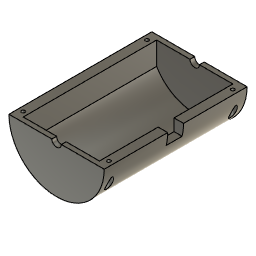
ShellTop (Autodesk Fusion 360 design; units mm, degrees)
Autodesk Fusion 360 part; units mm, degrees
note: some values were not read from the file. Set by a fixed rule: which sketch regions a step uses.
sketch "Sketch1" plane through (0, 0, 0) normal (0, 1, 0) x (1, 0, 0)
  circle A0 centre (38.1, -38.1) radius 38.1
  circle A1 centre (38.1, -38.1) radius 35.56
  circle A2 centre (38.1, -38.1) radius 3.81
  line L0 (38.1, -38.1) -> (0, -38.1)
  line L1 (38.1, -38.1) -> (76.2, -38.1)
  dimension "d1" = 76.2
  dimension "d2" = 71.12
  dimension "d4" = 7.62
  constraint concentric A0 A1
  constraint concentric A0 A2
  constraint coincident A0.centre A1.centre
  constraint coincident A0 L0.end
  constraint horizontal L0
  constraint coincident A0 L1.end
  constraint parallel L0 L1
  measures "d1" diameter of A0
  measures "d2" diameter of A1
  measures "d4" diameter of A2
extrude "Extrude1" add sketch "Sketch1" along normal blind 3.81 contours A1 A2 L0 L1 picked at (13.2699, -36.1441) makes body 1
extrude "Extrude2" add sketch "Sketch1" along normal blind 3.81 from surface at 110.49 separate body contours A1 A2 L0 L1 picked at (13.2699, -36.1441) makes body 2
extrude "Extrude3" add sketch "Sketch1" along normal blind 114.3 contours A0 A1 L0 L1 picked at (75.2115, -36.2072) bodies 1 2
sketch "Sketch2" plane through (0, 0, 38.1) normal (0, 0, 1) x (-1, 0, 0)
  line L0 (0, 0) -> (-34.29, 0)
  line L1 (-34.29, 0) -> (-34.29, -3.81)
  line L2 (-34.29, -3.81) -> (-2.54, -3.81)
  line L3 (-2.54, -3.81) -> (-2.54, -110.49)
  line L4 (-2.54, -110.49) -> (-34.29, -110.49)
  line L5 (-34.29, -110.49) -> (-34.29, -114.3)
  line L6 (-34.29, -114.3) -> (0, -114.3)
  line L7 (0, -114.3) -> (0, 0)
  line L8 (0, 0) -> (-7.62, 0)
  line L9 (-7.62, 0) -> (-7.62, -114.3)
  line L10 (-7.62, -114.3) -> (0, -114.3)
  line L11 (0, -114.3) -> (0, 0)
  line L12 (-76.2, 0) -> (-68.58, 0)
  line L13 (-68.58, 0) -> (-68.58, -114.3)
  line L14 (-68.58, -114.3) -> (-76.2, -114.3)
  line L15 (-76.2, -114.3) -> (-76.2, 0)
  dimension "d12" = 7.62
  dimension "d13" = 7.62
  constraint horizontal L8
  constraint vertical L9
  constraint horizontal L10
  constraint vertical L11
  constraint coincident L0.start L7.end
  constraint horizontal L12
  constraint vertical L13
  constraint horizontal L14
  constraint vertical L15
  measures "d12" distance of L0.start L8.end
  measures "d13" distance of L12.start L12.end
extrude "Extrude4" add sketch "Sketch2" against normal blind 27.94 contours L0 L2 L3 L4 L6 L7 L8 L9 L10 L11 | L2 L3 L4 L9 | L12 L13 L14 L15 bodies 1
extrude "Extrude5" cut sketch "Sketch1" along normal blind 121.92 contours A0 A1 L0 L1 | A1 A2 L0 L1 picked at (75.2115, -36.2072) picked at (13.2699, -36.1441) keep common part bodies 1
sketch "Sketch3" plane through (0, 0, 38.1) normal (0, 0, 1) x (-1, 0, 0)
  line L0 (0, 0) -> (-34.29, 0)
  line L1 (-34.29, 0) -> (-34.29, -3.81)
  line L2 (-34.29, -3.81) -> (-7.62, -3.81)
  line L3 (-7.62, -3.81) -> (-7.62, -110.49)
  line L4 (-7.62, -110.49) -> (-34.29, -110.49)
  line L5 (-34.29, -110.49) -> (-34.29, -114.3)
  line L6 (-34.29, -114.3) -> (0, -114.3)
  line L7 (0, -114.3) -> (0, 0)
  circle A0 centre (-3.81, -7.62) radius 2.54
  circle A1 centre (-3.81, -7.62) radius 1.397
  circle A2 centre (-72.39, -7.62) radius 1.397
  circle A3 centre (-72.39, -7.62) radius 2.54
  circle A4 centre (-3.81, -106.68) radius 1.397
  circle A5 centre (-3.81, -106.68) radius 2.54
  circle A6 centre (-72.39, -106.68) radius 1.397
  circle A7 centre (-72.39, -106.68) radius 2.54
  dimension "d18" = 5.08
  dimension "d19" = 7.62
  dimension "d20" = 2.794
  dimension "d23" = -68.58
  dimension "d24" = -99.06
  constraint concentric A0 A1
  measures "d18" diameter of A0
  measures "d19" distance of L0 A0.centre
  measures "d20" diameter of A1
extrude "Extrude6" cut sketch "Sketch3" against normal blind 43.18 contours A1 | A2 | A4 | A6 bodies 1
extrude "Extrude7" cut sketch "Sketch3" against normal blind 25.4 from surface at -2.54 contours A0 | A3 | A5 | A7 bodies 1
sketch "Sketch4" plane through (68.58, 0, 0) normal (-1, 0, 0) x (0, -1, 0)
  line L0 (-3.81, 19.7838) -> (-3.81, 38.1)
  line L1 (-3.81, 38.1) -> (-110.49, 38.1)
  line L2 (-110.49, 38.1) -> (-110.49, 19.7838)
  line L3 (-110.49, 19.7838) -> (-3.81, 19.7838)
  line L4 (-50.8, 38.1) -> (-63.5, 38.1)
  line L5 (-63.5, 38.1) -> (-63.5, 28.575)
  line L6 (-63.5, 28.575) -> (-50.8, 28.575)
  line L7 (-50.8, 28.575) -> (-50.8, 38.1)
  line L8 (0, 38.1) -> (0, 0)
  dimension "d30" = 12.7
  dimension "d31" = 50.8
  dimension "d32" = 9.525
  constraint horizontal L4
  constraint vertical L5
  constraint horizontal L6
  constraint vertical L7
  constraint coincident L1 L4.start
  measures "d30" distance of L5 L7
  measures "d31" distance of L7 L8
  measures "d32" distance of L4.end L5.end
extrude "Extrude8" cut sketch "Sketch4" against normal blind 7.62 contours L1 L4 L5 L6 L7 bodies 1
